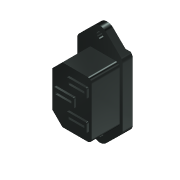
# Autodesk Inventor part: PlugFemeaTomada
Saved by Autodesk Inventor 2020 (Build 240168000, 168)
## iProperties
Created: 2015-09-19
Part Number: PlugFemeaTomada
Material: Plastic, Opaque Black
Document SubType Name: Modeling
Designer: Elvis Mayk
Density: 0.952 g/cm^3
Appearance: Gunmetal - Polished
Author: Elvis Mayk
Autodesk Inventor part; units mm, degrees
ref_plane "YZ Plane" through (0, 0, 0) normal (1, 0, 0) x (0, 1, 0)
ref_plane "XZ Plane" through (0, 0, 0) normal (0, 1, 0) x (-1, 0, 0)
ref_plane "XY Plane" through (0, 0, 0) normal (0, 0, 1) x (1, 0, 0)
sketch "Sketch1" plane through (0, 0, 0) normal (0, 1, 0) x (-1, 0, 0)
  arc A0 (2.8034, 23.3533) -> (-2.8034, 23.3533) centre (0, 20.5) ccw
  line L0 (-11, 14.0418) -> (-11, 0)
  line L1 (11, 14.0418) -> (11, 0)
  line L2 (11, 0) -> (-11, 0)
  line L3 (10.1025, 16.1818) -> (2.8034, 23.3533)
  line L4 (-10.1025, 16.1818) -> (-2.8034, 23.3533)
  arc A1 (11, 14.0418) -> (10.1025, 16.1818) centre (8, 14.0418) ccw
  arc A2 (-10.1025, 16.1818) -> (-11, 14.0418) centre (-8, 14.0418) ccw
  arc A3 (-2.8034, -23.3533) -> (2.8034, -23.3533) centre (0, -20.5) ccw
  line L5 (-11, -14.0418) -> (-11, 0)
  line L6 (11, -14.0418) -> (11, 0)
  line L7 (10.1025, -16.1818) -> (2.8034, -23.3533)
  line L8 (-10.1025, -16.1818) -> (-2.8034, -23.3533)
  arc A4 (10.1025, -16.1818) -> (11, -14.0418) centre (8, -14.0418) ccw
  arc A5 (-11, -14.0418) -> (-10.1025, -16.1818) centre (-8, -14.0418) ccw
  point P0 (0, 0)
  point P1 (11, 15.3)
  point P2 (-11, 15.3)
  point P3 (11, -15.3)
  point P4 (-11, -15.3)
  dimension "d0" = 0
  dimension "d1" = 22
  dimension "d2" = 11
  dimension "d3" = 8
  dimension "d4" = 15.3
  dimension "d5" = 0
  dimension "d6" = 15.3
  dimension "d7" = 20.5
  dimension "d8" = 3
  constraints: 18 end point, 12 point on circle, 11 symmetric about line, 8 point on line, 6 centre point, 6 tangent, 1 equal radius, 1 horizontal, 1 vertical, 3 other
  measures "d0" horizontal distance of A0.centre point (0, 0)
  measures "d1" distance between parallel lines of L0 L1
  measures "d2" distance from line of point (0, 0) L1
  measures "d3" diameter of A0
  measures "d4" distance of point (11, 15.3) L1.end
  measures "d5" vertical distance of point (0, 0) L1.end
  measures "d6" distance of point (-11, 15.3) L0.end
  measures "d7" distance of A0.centre point (0, 0)
  measures "d8" radius of A1
extrude "Extrusion1" add sketch "Sketch1" along normal blind 4.8
sketch "Sketch2" plane through (0, 4.8, 0) normal (0, 1, 0) x (1, 0, 0)
  line L0 (-10.1025, -16.1818) -> (-2.8034, -23.3533) projected
  line L1 (2.8034, -23.3533) -> (10.1025, -16.1818) projected
  line L2 (-10.1025, -16.1818) -> (10.1025, -16.1818)
  line L3 (-2.8034, 23.3533) -> (-10.1025, 16.1818) projected
  line L4 (10.1025, 16.1818) -> (2.8034, 23.3533) projected
  line L5 (-10.1025, 16.1818) -> (10.1025, 16.1818)
  arc A0 (-2.8034, -23.3533) -> (2.8034, -23.3533) centre (0, -20.5) ccw projected
  arc A1 (2.8034, 23.3533) -> (-2.8034, 23.3533) centre (0, 20.5) ccw projected
  point P0 (0, 0)
  constraints: 5 end point, 2 horizontal
extrude "Extrusion2" cut sketch "Sketch2" against normal blind 1.3
sketch "Sketch3" plane through (0, 3.5, 0) normal (0, 1, 0) x (1, 0, 0)
  arc A0 (-2.8034, -23.3533) -> (2.8034, -23.3533) centre (0, -20.5) ccw projected
  point P0 (0, 0)
  point P1 (0, 20.5)
  constraints: 1 coincident
hole "Hole1" at (0, 3.5, 20.5) at (0, 3.5, -20.5) direction (0, -1, 0) diameter 3.2 depth 8 tip angle 118 countersink diameter 5.7 countersink angle 90
sketch "Sketch5" plane through (0, 0, 0) normal (0, -1, 0) x (1, 0, 0)
  line L0 (7.5, -13.55) -> (-4.7, -13.55)
  line L1 (-9.5, -8.75) -> (-9.5, 8.75)
  line L2 (-4.7, 13.55) -> (7.5, 13.55)
  line L3 (9.5, 11.55) -> (9.5, -11.55)
  line L4 (9.5, -13.55) -> (-9.5, 13.55) construction
  line L5 (-9.5, -13.55) -> (9.5, 13.55) construction
  line L6 (-9.5, -8.75) -> (-4.7, -13.55)
  line L7 (-9.5, 8.75) -> (-4.7, 13.55)
  arc A0 (7.5, -13.55) -> (9.5, -11.55) centre (7.5, -11.55) ccw
  arc A1 (9.5, 11.55) -> (7.5, 13.55) centre (7.5, 11.55) ccw
  point P0 (0, 0)
  dimension "d20" = 4.8
  dimension "d21" = 4.8
  dimension "d22" = 4.8
  dimension "d23" = 4.8
  dimension "d24" = 19
  dimension "d25" = 2
  dimension "d26" = 27.1
  constraints: 16 end point, 8 point on line, 4 point on circle, 4 tangent, 2 centre point, 2 midpoint, 2 parallel, 1 equal radius, 1 horizontal, 1 perpendicular
  measures "d20" distance of L1.start L5.start
  measures "d21" distance of L0.end L5.start
  measures "d22" distance of L1.end L4.end
  measures "d23" distance of L2.start L4.end
  measures "d24" distance between parallel lines of L3 L1
  measures "d25" radius of A0
  measures "d26" distance between parallel lines of L2 L0
extrude "Extrusion3" add sketch "Sketch5" along normal blind 13.5
sketch "Sketch6" plane through (0, 4.8, 0) normal (0, 1, 0) x (1, 0, 0)
  line L0 (6.13, -12.15) -> (-3.13, -12.15)
  line L1 (-8.13, -7.15) -> (-8.13, 7.15)
  line L2 (-3.13, 12.15) -> (6.13, 12.15)
  line L3 (8.13, 10.15) -> (8.13, -10.15)
  line L4 (8.13, -12.15) -> (-8.13, 12.15) construction
  line L5 (-8.13, -12.15) -> (8.13, 12.15) construction
  arc A0 (6.13, -12.15) -> (8.13, -10.15) centre (6.13, -10.15) ccw
  arc A1 (8.13, 10.15) -> (6.13, 12.15) centre (6.13, 10.15) ccw
  line L6 (-8.13, -7.15) -> (-3.13, -12.15)
  line L7 (-8.13, 7.15) -> (-3.13, 12.15)
  point P0 (0, 0)
  dimension "d29" = 2
  dimension "d30" = 24.3
  dimension "d31" = 16.26
  dimension "d32" = 5
  dimension "d33" = 45
  dimension "d34" = 5
  dimension "d35" = 45
  constraints: 16 end point, 8 point on line, 4 point on circle, 4 tangent, 2 centre point, 2 midpoint, 2 parallel, 1 equal radius, 1 horizontal, 1 perpendicular
  measures "d29" radius of A0
  measures "d30" distance between parallel lines of L2 L0
  measures "d31" distance between parallel lines of L3 L1
  measures "d32" distance of L1.start L5.start
  measures "d33" angle of L1 L6
  measures "d34" distance of L1.end L4.end
  measures "d35" angle of L1 L7
extrude "Extrusion4" cut sketch "Sketch6" against normal blind 17.5
sketch "Sketch7" plane through (0, -13.5, 0) normal (0, -1, 0) x (1, 0, 0)
  line L0 (1.4, -2.3) -> (-7.6, -2.3)
  line L1 (-8.1, -1.8) -> (-8.1, 1.8)
  line L2 (-7.6, 2.3) -> (1.4, 2.3)
  line L3 (1.9, 1.8) -> (1.9, -1.8)
  line L4 (1.9, -2.3) -> (-8.1, 2.3) construction
  line L5 (-8.1, -2.3) -> (1.9, 2.3) construction
  line L6 (7.6, -9.5) -> (-1.4, -9.5)
  line L7 (-1.9, -9) -> (-1.9, -5.4)
  line L8 (-1.4, -4.9) -> (7.6, -4.9)
  line L9 (8.1, -5.4) -> (8.1, -9)
  line L10 (8.1, -9.5) -> (-1.9, -4.9) construction
  line L11 (-1.9, -9.5) -> (8.1, -4.9) construction
  line L12 (-9.5, -8.75) -> (-4.7, -13.55) projected
  line L13 (-4.7, -13.55) -> (7.5, -13.55) projected
  arc A0 (7.5, -13.55) -> (9.5, -11.55) centre (7.5, -11.55) ccw projected
  line L14 (9.5, -11.55) -> (9.5, 11.55) projected
  arc A1 (9.5, 11.55) -> (7.5, 13.55) centre (7.5, 11.55) ccw projected
  line L15 (7.5, 13.55) -> (-4.7, 13.55) projected
  line L16 (-4.7, 13.55) -> (-9.5, 8.75) projected
  line L17 (-9.5, 8.75) -> (-9.5, -8.75) projected
  line L18 (-9.5, 0) -> (9.5, 0)
  arc A2 (-8.1, -1.8) -> (-7.6, -2.3) centre (-7.6, -1.8) ccw
  arc A3 (-7.6, 2.3) -> (-8.1, 1.8) centre (-7.6, 1.8) ccw
  arc A4 (1.9, 1.8) -> (1.4, 2.3) centre (1.4, 1.8) ccw
  arc A5 (1.4, -2.3) -> (1.9, -1.8) centre (1.4, -1.8) ccw
  arc A6 (-1.4, -4.9) -> (-1.9, -5.4) centre (-1.4, -5.4) ccw
  arc A7 (8.1, -5.4) -> (7.6, -4.9) centre (7.6, -5.4) ccw
  arc A8 (7.6, -9.5) -> (8.1, -9) centre (7.6, -9) ccw
  arc A9 (-1.9, -9) -> (-1.4, -9.5) centre (-1.4, -9) ccw
  line L19 (7.6, 9.5) -> (-1.4, 9.5)
  line L20 (-1.9, 9) -> (-1.9, 5.4)
  line L21 (-1.4, 4.9) -> (7.6, 4.9)
  line L22 (8.1, 5.4) -> (8.1, 9)
  line L23 (8.1, 9.5) -> (-1.9, 4.9) construction
  line L24 (-1.9, 9.5) -> (8.1, 4.9) construction
  arc A10 (-1.9, 5.4) -> (-1.4, 4.9) centre (-1.4, 5.4) ccw
  arc A11 (7.6, 4.9) -> (8.1, 5.4) centre (7.6, 5.4) ccw
  arc A12 (8.1, 9) -> (7.6, 9.5) centre (7.6, 9) ccw
  arc A13 (-1.4, 9.5) -> (-1.9, 9) centre (-1.4, 9) ccw
  point P0 (0, 0)
  point P1 (-3.1, 0)
  point P2 (3.1, -7.2)
  point P3 (3.1, 7.2)
  dimension "d38" = 10
  dimension "d39" = 4.6
  dimension "d40" = 2.6
  dimension "d41" = 10
  dimension "d42" = 4.6
  dimension "d43" = 0.5
  dimension "d44" = 1.4
  dimension "d45" = 1.4
  constraints: 38 end point, 25 point on line, 24 point on circle, 17 symmetric about line, 16 tangent, 12 centre point, 8 midpoint, 7 equal radius, 4 parallel, 2 horizontal, 2 perpendicular, 4 other
  measures "d38" distance of L4.end L5.end
  measures "d39" distance of L5.start L4.end
  measures "d40" distance between parallel lines of L0 L8
  measures "d41" distance of L10.start L11.start
  measures "d42" distance of L11.start L10.end
  measures "d43" radius of A2
  measures "d44" distance between parallel lines of L14 L9
  measures "d45" distance between parallel lines of L17 L1
extrude "Extrusion5" add sketch "Sketch7" along normal blind 1 contours L0 A2 L1 L18 L3 A5 | L18 L1 A3 L2 A4 L3 | L6 A9 L7 A6 L8 A7 L9 A8 | A12 L22 A11 L21 A10 L20 A13 L19
sketch "Sketch8" plane through (0, -14.5, 0) normal (0, -1, 0) x (1, 0, 0)
  line L0 (-7.6, -2.3) -> (1.4, -2.3) projected
  arc A0 (1.4, -2.3) -> (1.9, -1.8) centre (1.4, -1.8) ccw projected
  line L1 (1.9, -1.8) -> (1.9, 1.8) projected
  arc A1 (1.9, 1.8) -> (1.4, 2.3) centre (1.4, 1.8) ccw projected
  line L2 (1.4, 2.3) -> (-7.6, 2.3) projected
  arc A2 (-7.6, 2.3) -> (-8.1, 1.8) centre (-7.6, 1.8) ccw projected
  line L3 (-8.1, 1.8) -> (-8.1, -1.8) projected
  arc A3 (-8.1, -1.8) -> (-7.6, -2.3) centre (-7.6, -1.8) ccw projected
  line L4 (7.6, -4.9) -> (-1.4, -4.9) projected
  arc A4 (-1.4, -4.9) -> (-1.9, -5.4) centre (-1.4, -5.4) ccw projected
  line L5 (-1.9, -5.4) -> (-1.9, -9) projected
  arc A5 (-1.9, -9) -> (-1.4, -9.5) centre (-1.4, -9) ccw projected
  line L6 (-1.4, -9.5) -> (7.6, -9.5) projected
  arc A6 (7.6, -9.5) -> (8.1, -9) centre (7.6, -9) ccw projected
  line L7 (8.1, -9) -> (8.1, -5.4) projected
  arc A7 (8.1, -5.4) -> (7.6, -4.9) centre (7.6, -5.4) ccw projected
  line L8 (-1.9, 9) -> (-1.9, 5.4) projected
  arc A8 (-1.9, 5.4) -> (-1.4, 4.9) centre (-1.4, 5.4) ccw projected
  line L9 (-1.4, 4.9) -> (7.6, 4.9) projected
  arc A9 (7.6, 4.9) -> (8.1, 5.4) centre (7.6, 5.4) ccw projected
  line L10 (8.1, 5.4) -> (8.1, 9) projected
  arc A10 (8.1, 9) -> (7.6, 9.5) centre (7.6, 9) ccw projected
  line L11 (7.6, 9.5) -> (-1.4, 9.5) projected
  arc A11 (-1.4, 9.5) -> (-1.9, 9) centre (-1.4, 9) ccw projected
  line L12 (-8.1, 1.8) -> (-8.1, -1.8) projected
  line L13 (-8.1, 0) -> (1.9, 0)
  line L14 (-7.6, -2.3) -> (1.4, -2.3) projected
  line L15 (-3.1, -2.3) -> (-3.1, 2.3)
  line L16 (-1.9, -5.4) -> (-1.9, -9) projected
  line L17 (-1.9, -7.2) -> (8.1, -7.2)
  line L18 (7.6, -9.5) -> (-1.4, -9.5) projected
  line L19 (3.1, -9.5) -> (3.1, -4.9)
  line L20 (7.6, -4.9) -> (-1.4, -4.9) projected
  line L21 (3.1, 4.9) -> (3.1, 9.5)
  line L22 (-1.9, 9) -> (-1.9, 5.4) projected
  line L23 (-1.9, 7.2) -> (8.1, 7.2)
  line L24 (6.9, -7.7) -> (-0.7, -7.7)
  line L25 (-0.7, -7.7) -> (-0.7, -6.7)
  line L26 (-0.7, -6.7) -> (6.9, -6.7)
  line L27 (6.9, -6.7) -> (6.9, -7.7)
  line L28 (6.9, -7.7) -> (-0.7, -6.7) construction
  line L29 (-0.7, -7.7) -> (6.9, -6.7) construction
  line L30 (0.7, -0.5) -> (-6.9, -0.5)
  line L31 (-6.9, -0.5) -> (-6.9, 0.5)
  line L32 (-6.9, 0.5) -> (0.7, 0.5)
  line L33 (0.7, 0.5) -> (0.7, -0.5)
  line L34 (0.7, -0.5) -> (-6.9, 0.5) construction
  line L35 (-6.9, -0.5) -> (0.7, 0.5) construction
  line L36 (6.9, 6.7) -> (-0.7, 6.7)
  line L37 (-0.7, 6.7) -> (-0.7, 7.7)
  line L38 (-0.7, 7.7) -> (6.9, 7.7)
  line L39 (6.9, 7.7) -> (6.9, 6.7)
  line L40 (6.9, 6.7) -> (-0.7, 7.7) construction
  line L41 (-0.7, 6.7) -> (6.9, 7.7) construction
  point P0 (0, 0)
  point P1 (3.1, -7.2)
  point P2 (-3.1, 0)
  point P3 (3.1, 7.2)
  dimension "d48" = 7.6
  dimension "d49" = 7.6
  dimension "d50" = 7.6
  dimension "d52" = 1
  dimension "d53" = 1
  dimension "d54" = 1
  constraints: 48 end point, 21 midpoint, 6 parallel, 3 horizontal, 3 perpendicular
  measures "d48" distance of L31.end L32.end
  measures "d49" distance of L25.end L26.end
  measures "d50" distance of L37.end L38.end
  measures "d52" distance of L30.end L31.end
  measures "d53" distance of L24.end L25.end
  measures "d54" distance of L36.end L37.end
extrude "Extrusion6" cut sketch "Sketch8" against normal through all contours L30 L31 L13 L15 | L15 L13 L33 L30 | L15 L32 L33 L13 | L13 L31 L32 L15 | L26 L27 L17 L19 | L19 L17 L25 L26 | L19 L24 L25 L17 | L17 L27 L24 L19 | L37 L38 L21 L23 | L23 L21 L36 L37 | L23 L39 L36 L21 | L21 L38 L39 L23
sketch "Sketch9" plane through (0, 3.5, 0) normal (0, 1, 0) x (1, 0, 0)
  circle A0 centre (0, 20.5) radius 1.6 projected
  circle A1 centre (0, 20.5) radius 0.2629
  circle A2 centre (0, 20) radius 1.625
  line L0 (0, 20) -> (0, -20)
  circle A3 centre (0, -20) radius 1.625
  point P0 (0, 0)
  point P1 (-1.591, 20.3306)
  point P2 (1.591, 20.3306)
  dimension "d57" = 3.25
  dimension "d58" = 0.5
  dimension "d61" = 40
  dimension "d62" = 3.25
  constraints: 3 centre point, 2 coincident, 2 end point, 1 vertical
  measures "d57" diameter of A2
  measures "d58" distance of A1.centre L0.start
  measures "d61" distance of L0.start L0.end
  measures "d62" diameter of A3
extrude "Extrusion7" cut sketch "Sketch9" against normal blind 10 contours A3 | A0 L0 A2 | A2 L0 A0
equation "\"d2\" = 0.5 * d1"
equation "\"d6\" = d4"
equation "\"d21\" = d20"
equation "\"d22\" = d20"
equation "\"d23\" = d22"
equation "\"d34\" = d32"
equation "\"d35\" = d33"
equation "\"d42\" = d39"
equation "\"d49\" = d48"
equation "\"d50\" = d48"
equation "\"d53\" = d52"
equation "\"d54\" = d52"
body "Solid1"
